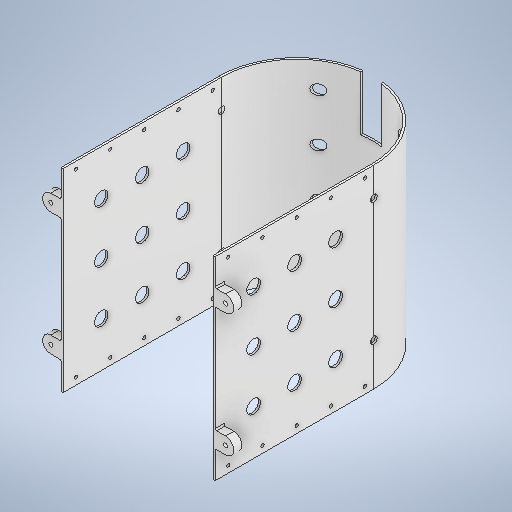
# Autodesk Inventor part: 1 part 05
Saved by Autodesk Inventor 2025.1 (Build 291241000, 241)
## iProperties
Created: 2024-07-30
Part Number: 1 part 05
Material: Acetalharz, Weiß
Document SubType Name: Modeling
Designer: ffogue
Density: 1.425 g/cm^3
Appearance: Glatt - Weiß
Author: ffogue
Autodesk Inventor part; units mm, degrees
ref_plane "YZ Plane" through (0, 0, 0) normal (1, 0, 0) x (0, 1, 0)
ref_plane "XY Plane" through (0, 0, 0) normal (0, 0, 1) x (1, 0, 0)
sketch "Skizze1" plane through (0, 0, 0) normal (0, 0, 1) x (1, 0, 0)
  line L0 (-55, 0) -> (-55, 116)
  arc A0 (55, 116) -> (-55, 116) centre (0, 116) ccw
  line L1 (55, 116) -> (55, 0)
  line L2 (-56.5, 0) -> (-56.5, 116)
  arc A1 (56.5, 116) -> (-56.5, 116) centre (0, 116) ccw
  line L3 (56.5, 116) -> (56.5, 0)
  line L4 (-55, 0) -> (-56.5, 0)
  line L5 (56.5, 0) -> (55, 0)
  line L6 (0, 0) -> (0, 86.7661) construction
  dimension "d0" = 1.5
  dimension "d1" = 110
  dimension "d2" = 116
  constraints: 14 end point, 4 point on circle, 3 horizontal alignment, 2 centre point, 2 parallel, 2 perpendicular, 2 vertical, 1 tangent, 1 vertical alignment, 3 other
  measures "d0" distance between parallel lines of L0 L2
  measures "d1" distance between parallel lines of L1 L0
  measures "d2" vertical distance of L0.start A0.centre
extrude "Extrusion1" add sketch "Skizze1" along normal mid plane 142
ref_plane "Arbeitsebene1" through (0, 173, 0) normal (0, 1, 0) x (-1, 0, 0)
sketch "Skizze2" plane through (0, 173, 0) normal (0, 1, 0) x (-1, 0, 0)
  line L0 (56.5, -71) -> (56.5, 71) projected
  line L1 (-56.5, 71) -> (56.5, 71) projected
  line L2 (-56.5, -71) -> (-56.5, 71) projected
  line L3 (56.5, -71) -> (-56.5, -71) projected
  line L4 (7.5, 71) -> (7.5, 31)
  line L5 (7.5, 31) -> (-7.5, 31)
  line L6 (-7.5, 31) -> (-7.5, 71)
  circle A0 centre (0, -40) radius 7.5
  circle A1 centre (0, -2) radius 7.5
  point P0 (0, 0)
  point P1 (0, 31)
  dimension "d6" = 40
  dimension "d7" = 15
  dimension "d8" = 15
  dimension "d9" = 15
  dimension "d10" = 31
  dimension "d11" = 38
  constraints: 6 end point, 3 vertical alignment, 2 centre point, 2 perpendicular, 2 point on line, 1 midpoint, 1 vertical
  measures "d6" distance between parallel lines of L5 L1
  measures "d7" distance between parallel lines of L6 L4
  measures "d8" diameter of A1
  measures "d9" diameter of A0
  measures "d10" distance from line of L3 A0.centre
  measures "d11" distance of A1.centre A0.centre
extrude "Extrusion2" cut sketch "Skizze2" against normal up to surface contours L4 L5 L6 L1 | A0 | A1
sketch "Skizze3" plane through (0, 173, 0) normal (0, 1, 0) x (-1, 0, 0)
  circle A0 centre (-30, 52.5) radius 3.75
  circle A1 centre (-30, 17.5) radius 3.75
  circle A2 centre (-30, -17.5) radius 3.75
  circle A3 centre (-30, -52.5) radius 3.75
  line L0 (-7.5, 71) -> (-56.5, 71) projected
  point P0 (0, 0)
  dimension "d14" = 30
  dimension "d15" = 7.5
  dimension "d16" = 18.5
  dimension "d17" = 35
  dimension "d18" = 35
  dimension "d19" = 35
  constraints: 4 centre point, 3 equal radius, 3 vertical alignment
  measures "d14" horizontal distance of A0.centre point (0, 0)
  measures "d15" diameter of A0
  measures "d16" distance from line of L0 A0.centre
  measures "d17" distance of A1.centre A0.centre
  measures "d18" distance of A2.centre A1.centre
  measures "d19" distance of A3.centre A2.centre
extrude "Extrusion3" cut sketch "Skizze3" against normal up to surface
mirror "Spiegeln1" about plane through (0, 0, 0) normal (1, 0, 0) of "Extrusion3"
sketch "Skizze4" plane through (56.5, 0, 71) normal (1, 0, 0) x (0, 0, -1)
  line L0 (142, 116) -> (0, 116) projected
  line L1 (142, 0) -> (0, 0) projected
  point P0 (71, 0)
  point P1 (21, 116)
  point P2 (111, 116)
  point P3 (71, 0)
  point P4 (71, 0)
  dimension "d22" = 50
  dimension "d23" = 40
  constraints: 2 horizontal alignment, 2 midpoint, 2 point on line
  measures "d22" horizontal distance of point (71, 0) point (21, 116)
  measures "d23" horizontal distance of point (71, 0) point (111, 116)
hole "Bohrung1" at (56.5, 116, 50) at (56.5, 116, -40) direction (-1, 0, 0) diameter 5 depth 1.5
mirror "Spiegeln2" about plane through (0, 0, 0) normal (1, 0, 0) of "Bohrung1"
sketch "Skizze5" plane through (56.5, 0, 71) normal (1, 0, 0) x (0, 0, -1)
  line L0 (0, 0) -> (0, 116) projected
  point P0 (71, 0)
  point P1 (33, 28)
  point P2 (33, 58)
  point P3 (33, 88)
  point P4 (71, 28)
  point P5 (71, 58)
  point P6 (71, 88)
  point P7 (109, 28)
  point P8 (109, 58)
  point P9 (109, 88)
  point P10 (0, 58)
  dimension "d31" = 38
  dimension "d32" = 38
  dimension "d33" = 33
  dimension "d34" = 30
  dimension "d35" = 30
  constraints: 7 horizontal alignment, 6 vertical alignment, 1 midpoint
  measures "d31" distance of point (71, 28) point (109, 28)
  measures "d32" distance of point (71, 28) point (33, 28)
  measures "d33" distance from line of L0 point (33, 28)
  measures "d34" distance of point (33, 58) point (33, 88)
  measures "d35" distance of point (33, 58) point (33, 28)
hole "Bohrung2" at (56.5, 28, 38) at (56.5, 58, 38) at (56.5, 88, 38) at (56.5, 28, 0) at (56.5, 58, 0) at (56.5, 88, 0) at (56.5, 28, -38) at (56.5, 58, -38) at (56.5, 88, -38) direction (-1, 0, 0) diameter 10 depth 1.5
mirror "Spiegeln3" about plane through (0, 0, 0) normal (1, 0, 0) of "Bohrung2"
sketch "Skizze6" plane through (-55, 0, -71) normal (0, -1, 0) x (1, 0, 0)
  line L0 (-1.5, 20) -> (-9, 20)
  line L1 (-9, 32) -> (-1.5, 32)
  line L2 (-1.5, 32) -> (-1.5, 20)
  line L3 (-1.5, 110) -> (-9, 110)
  line L4 (-9, 122) -> (-1.5, 122)
  line L5 (-1.5, 122) -> (-1.5, 110)
  arc A0 (-9, 32) -> (-9, 20) centre (-9, 26) ccw
  arc A1 (-9, 122) -> (-9, 110) centre (-9, 116) ccw
  line L6 (110, 0) -> (0, 0) projected
  line L7 (-1.5, 0) -> (-1.5, 142) projected
  point P0 (55, 71)
  point P1 (-1.5, 26)
  point P2 (-1.5, 116)
  dimension "d43" = 6
  dimension "d44" = 6
  dimension "d47" = 26
  dimension "d48" = 90
  dimension "d49" = 64
  constraints: 12 end point, 4 point on circle, 4 tangent, 2 centre point, 2 horizontal, 2 midpoint, 2 parallel, 2 point on line, 1 vertical alignment
  measures "d43" radius of A0
  measures "d44" radius of A1
  measures "d47" distance from line of L6 A0.centre
  measures "d48" distance of A1.centre A0.centre
  measures "d49" horizontal distance of A0.centre point (55, 71)
extrude "Extrusion4" add sketch "Skizze6" against normal blind 6
sketch "Skizze7" plane through (-55, 6, -71) normal (0, 1, 0) x (1, 0, 0)
  arc A0 (-9, -20) -> (-9, -32) centre (-9, -26) ccw projected
  arc A1 (-9, -110) -> (-9, -122) centre (-9, -116) ccw projected
  point P0 (55, -71)
  constraints: 2 coincident
hole "Bohrung3" at (-64, 6, -45) at (-64, 6, 45) direction (0, -1, 0) diameter 3 depth 6
fillet "Rundung1" radius 1 6 edges at (-56.5, 6, 45) (-56.5, 3, 39) (-56.5, 3, 51) (-56.5, 3, -39) (-56.5, 6, -45) (-56.5, 3, -51)
mirror "Spiegeln4" about plane through (0, 0, 0) normal (1, 0, 0) of "Extrusion4", "Rundung1", "Bohrung3"
sketch "Skizze8" plane through (-56.5, 0, 71) normal (-1, 0, 0) x (0, 0, 1)
  line L0 (-142, 0) -> (-123, 0) projected
  line L1 (-142, 0) -> (-142, 116) projected
  point P0 (-71, 0)
  point P1 (-137, 9.5)
  point P2 (-137, 34.5)
  point P3 (-137, 59.5)
  point P4 (-137, 84.5)
  point P5 (-137, 109.5)
  dimension "d60" = 9.5
  dimension "d61" = 25
  dimension "d62" = 25
  dimension "d63" = 25
  dimension "d64" = 25
  dimension "d65" = 5
  constraints: 4 vertical alignment
  measures "d60" distance from line of L0 point (-137, 9.5)
  measures "d61" distance of point (-137, 34.5) point (-137, 9.5)
  measures "d62" distance of point (-137, 59.5) point (-137, 34.5)
  measures "d63" distance of point (-137, 84.5) point (-137, 59.5)
  measures "d64" distance of point (-137, 109.5) point (-137, 84.5)
  measures "d65" distance from line of L1 point (-137, 109.5)
hole "Bohrung4" at (-56.5, 9.5, -66) at (-56.5, 34.5, -66) at (-56.5, 59.5, -66) at (-56.5, 84.5, -66) at (-56.5, 109.5, -66) direction (1, 0, 0) diameter 2.459 depth 1.5 thread size "M3x0.5" class "6H" standard "ISO Metric profile"
mirror "Spiegeln5" about plane through (0, 0, 0) normal (0, 0, 1) of "Bohrung4"
mirror "Spiegeln6" about plane through (0, 0, 0) normal (1, 0, 0) of "Bohrung4", "Spiegeln5"
equation "\"d18\" = d17"
equation "\"d19\" = d17"
equation "\"d32\" = d31"
equation "\"d62\" = d61"
equation "\"d63\" = d61"
equation "\"d64\" = d61"
